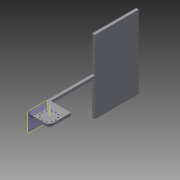
# Autodesk Inventor part: second_perc_link
Saved by Autodesk Inventor 2015 (Build 190159000, 159)
## iProperties
Created: 2014-10-20
Part Number: second_perc_link
Material: Generic
Document SubType Name: Modeling
Designer: ericd_000
Density: 1 g/cm^3
Appearance: Default
Author: ericd_000
Autodesk Inventor part; units mm, degrees
ref_plane "YZ Plane" through (0, 0, 0) normal (1, 0, 0) x (0, 1, 0)
ref_plane "XZ Plane" through (0, 0, 0) normal (0, 1, 0) x (-1, 0, 0)
ref_plane "XY Plane" through (0, 0, 0) normal (0, 0, 1) x (1, 0, 0)
sketch "Sketch1" plane through (0, 0, 0) normal (0, 0, 1) x (1, 0, 0)
  line L0 (-9, 25) -> (9, 25)
  line L1 (9, 25) -> (9, -25)
  line L2 (9, -25) -> (-9, -25)
  line L3 (-9, -25) -> (-9, 25)
  point P0 (0, 0)
  point P1 (0, 25)
  point P2 (-9, 0)
  dimension "d0" = 18
  dimension "d1" = 50
  constraints: 8 end point, 2 midpoint, 2 parallel, 1 horizontal, 1 horizontal alignment, 1 perpendicular, 1 vertical alignment
  measures "d0" distance of L1.end L2.end
  measures "d1" distance of L0.end L1.end
extrude "Extrusion1" add sketch "Sketch1" along normal blind 3
sketch "Sketch2" plane through (0, 0, 3) normal (0, 0, 1) x (1, 0, 0)
  circle A0 centre (0, -16) radius 9
  circle A1 centre (0, 16) radius 9
  line L0 (-9, -25) -> (9, -25) projected
  circle A2 centre (0, -8.304) radius 0.75
  line L1 (9, 25) -> (-9, 25) projected
  point P0 (0, 0)
  point P1 (-4, -25)
  point P2 (4, -25)
  point P3 (4, 25)
  point P4 (-4, 25)
  dimension "d6" = 18
  dimension "d8" = 1.5
  dimension "d10" = 18
  constraints: 3 centre point, 2 tangent
  measures "d6" diameter of A0
  measures "d8" diameter of A2
  measures "d10" diameter of A1
extrude "Extrusion2" cut sketch "Sketch2" against normal up to surface (3 mm away) contours A2
pattern_circular "Circular Pattern1" count 12 over 360 about axis through (0, -16, 3) along (0, 0, 1) of "Extrusion2"
sketch "Sketch7" plane through (0, 0, 3) normal (0, 0, 1) x (1, 0, 0)
  line L0 (-19, 0) -> (11, 0)
  line L1 (11, 0) -> (11, 28.3489)
  line L2 (11, 28.3489) -> (-19, 28.3489)
  line L3 (-19, 28.3489) -> (-19, 0)
  line L4 (-9, -25) -> (9, -25) projected
  line L5 (-9, 25) -> (-9, -25) projected
  line L6 (9, -25) -> (9, 25) projected
  point P0 (0, 0)
  point P1 (-4, -25)
  point P2 (4, -25)
  point P3 (-9, 20)
  point P4 (-9, -20)
  point P5 (9, -20)
  dimension "d44" = 25
  dimension "d48" = 30
  dimension "d49" = 2
  constraints: 8 end point, 2 parallel, 1 horizontal, 1 perpendicular
  measures "d44" distance between parallel lines of L4 L0
  measures "d48" distance of L1.end L2.end
  measures "d49" distance between parallel lines of L6 L1
extrude "Extrusion8" cut sketch "Sketch7" against normal up to surface (3 mm away) contours L3 L2 L1 L0
ref_plane "Work Plane1" through (-9, -20, 0) normal (-1, 0, 0) x (0, 0, 1)
sketch "Sketch9" plane through (-9, -20, 0) normal (-1, 0, 0) x (0, 0, 1)
  line L0 (3, 0) -> (3, 20)
  line L1 (3, 20) -> (0, 20)
  line L2 (0, 20) -> (0, 0)
  line L3 (3, 0) -> (3, -5)
  line L4 (3, -5) -> (0, -5)
  line L5 (0, -5) -> (3, -5) projected
  line L6 (0, -5) -> (0, 0)
  constraints: 12 end point, 2 equal length, 1 perpendicular, 1 vertical
extrude "Extrusion9" add sketch "Sketch9" along normal blind 8
fillet "Fillet3" radius 5 1 edges at (9, -25, 1.5)
sketch "Sketch10" plane through (9, 0, 3) normal (0, 1, 0) x (1, 0, 0)
  line L0 (-5, 3) -> (-26, 3) projected
  line L1 (-26, 0) -> (-23, 0)
  line L2 (-23, 0) -> (-23, 3)
  line L3 (-23, 3) -> (-26, 3)
  line L4 (-26, 3) -> (-26, 0)
  point P0 (-9, 3)
  dimension "d53" = 3
  constraints: 8 end point, 2 parallel, 1 horizontal, 1 perpendicular, 1 point on line
  measures "d53" distance of L1.start L1.end
extrude "Extrusion10" add sketch "Sketch10" along normal blind 70
fillet "Fillet4" radius 5 1 edges at (-17, -25, 1.5)
sketch "Sketch11" plane through (0, 0, 3) normal (0, 0, 1) x (1, 0, 0)
  line L0 (-14, 0) -> (-14, 70) projected
  line L1 (-17, 70) -> (-14, 70)
  line L2 (-14, 70) -> (-14, 50)
  line L3 (-14, 50) -> (-17, 50)
  line L4 (-17, 50) -> (-17, 70)
  point P0 (0, 0)
  dimension "d57" = 20
  constraints: 8 end point, 2 parallel, 1 horizontal, 1 perpendicular, 1 point on line
  measures "d57" distance of L3.end L1.start
extrude "Extrusion11" add sketch "Sketch11" along normal blind 30
sketch "Sketch12" plane through (0, 0, 0) normal (0, 0, -1) x (-1, 0, 0)
  line L0 (14, 0) -> (14, 70) projected
  line L1 (17, 70) -> (14, 70)
  line L2 (14, 70) -> (14, 50)
  line L3 (14, 50) -> (17, 50)
  line L4 (17, 50) -> (17, 70)
  point P0 (0, 0)
  dimension "d60" = 20
  constraints: 8 end point, 2 parallel, 1 horizontal, 1 perpendicular, 1 point on line
  measures "d60" distance of L3.end L1.start
extrude "Extrusion12" add sketch "Sketch12" along normal blind 30
sketch "Sketch13" plane through (9, 70, 3) normal (0, 1, 0) x (1, 0, 0)
  line L0 (-26, 33) -> (-23, 33)
  line L1 (-23, 33) -> (-23, -30)
  line L2 (-23, -30) -> (-26, -30)
  line L3 (-26, -30) -> (-26, 33)
  point P0 (-9, 3)
  constraints: 8 end point, 2 parallel, 1 horizontal, 1 perpendicular
extrude "Extrusion13" add sketch "Sketch13" along normal blind 30
sketch "Sketch14" plane through (0, 0, 33) normal (0, 0, 1) x (1, 0, 0)
  line L0 (-17, 50) -> (-14, 50)
  line L1 (-14, 50) -> (-14, 100)
  line L2 (-14, 100) -> (-17, 100)
  line L3 (-17, 100) -> (-17, 50)
  point P0 (0, 0)
  constraints: 8 end point, 2 parallel, 1 horizontal, 1 perpendicular
extrude "Extrusion14" add sketch "Sketch14" along normal blind 10
sketch "Sketch15" plane through (0, 0, -30) normal (0, 0, -1) x (-1, 0, 0)
  line L0 (17, 100) -> (14, 100)
  line L1 (14, 100) -> (14, 50)
  line L2 (14, 50) -> (17, 50)
  line L3 (17, 50) -> (17, 100)
  point P0 (0, 0)
  constraints: 8 end point, 2 parallel, 1 horizontal, 1 perpendicular
extrude "Extrusion15" add sketch "Sketch15" along normal blind 10
body "Solid1"
